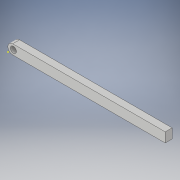
# Autodesk Inventor part: RoboArm 2020 Arm
Saved by Autodesk Inventor 2019 (Build 230136000, 136)
## iProperties
Created: 2020-02-03
Part Number: RoboArm 2020 Arm
Material: Generic
Document SubType Name: Modeling
Designer: mbird
Density: 1 g/cm^3
Appearance: Default
Author: mbird
Autodesk Inventor part; units mm, degrees
ref_plane "YZ Plane" through (0, 0, 0) normal (1, 0, 0) x (0, 1, 0)
ref_plane "XZ Plane" through (0, 0, 0) normal (0, 1, 0) x (-1, 0, 0)
ref_plane "XY Plane" through (0, 0, 0) normal (0, 0, 1) x (1, 0, 0)
sketch "Sketch3" plane through (0, 0, 0) normal (0, 0, 1) x (1, 0, 0)
  line L0 (0, 0) -> (570, 0)
  line L1 (570, 0) -> (570, 35)
  line L2 (570, 35) -> (0, 35)
  line L3 (0, 35) -> (0, 0)
  dimension "d3" = 570
  dimension "d4" = 35
  constraints: 8 end point, 2 parallel, 1 horizontal, 1 perpendicular
  measures "d3" distance of L2.end L1.end
  measures "d4" distance of L1.end L0.end
extrude "Extrusion2" add sketch "Sketch3" along normal blind 25
sketch "Sketch4" plane through (0, 0, 25) normal (0, 0, 1) x (1, 0, 0)
  point P0 (0, 0)
sketch "Sketch5" plane through (0, 0, 25) normal (0, 0, 1) x (1, 0, 0)
  line L0 (0, 35) -> (0, 0) projected
  point P0 (20, 17.5)
hole "Hole1" at (20, 17.5, 25) direction (0, 0, -1) diameter 22 end through all
fillet "Fillet4" radius 17.5 1 edges at (0, 35, 12.5)
fillet "Fillet5" radius 17.5 1 edges at (0, 0, 12.5)
body "Solid2"
